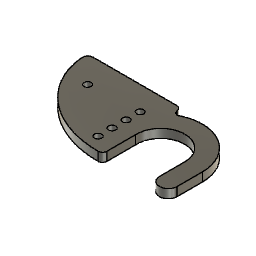
Hook v1 (Autodesk Fusion 360 design; units mm, degrees)
Autodesk Fusion 360 part; units mm, degrees
sketch "Sketch1" plane through (0, 0, 0) normal (0, 0, 1) x (1, 0, 0)
  line L0 (-13.7051, 19.3551) -> (-13.7051, 25.547)
  line L1 (-13.7051, 0.547) -> (-13.7051, -19.453)
  line L2 (-13.7051, -19.453) -> (-105.7051, -19.453)
  line L3 (-13.7051, 25.547) -> (-105.7051, 25.547)
  line L4 (-105.7051, 25.547) -> (-105.7051, -19.453)
  line L5 (13.716, -0.005) -> (13.716, -14.405)
  line L6 (23.716, 0.0066) -> (23.716, -14.3934)
  arc A0 (23.716, 0.0066) -> (-13.7051, 19.3551) centre (0, 0) ccw
  arc A1 (13.716, -0.005) -> (-13.7051, -0.547) centre (0, 0) ccw
  line L7 (13.716, -14.405) -> (23.716, -14.3934)
  circle A2 centre (18.716, -14.3992) radius 5
  dimension "d1" = 27.432
  dimension "d2" = 47.432
  dimension "d4" = 25
  dimension "d5" = 20
  dimension "d6" = 92
  dimension "d7" = 92
  dimension "d8" = 14.4
  dimension "d9" = 14.4
  dimension "d60" = 10
  constraint coincident A0.centre A1.centre
  constraint concentric A0 A1
  constraint coincident L1.start A1
  constraint parallel L0 L1
  constraint perpendicular L1 L2
  constraint perpendicular L0 L3
  constraint vertical L5
  constraint vertical L6
  constraint coincident L1 A1.end
  constraint midpoint L7 A2.centre
  constraint coincident L6.end A2
  measures "d1" diameter of A1
  measures "d2" diameter of A0
  measures "d4" distance of L1.start L0.end
  measures "d5" distance of L1.start L1.end
  measures "d6" distance of L1.end L2.end
  measures "d7" distance of L0.end L3.end
  measures "d8" distance of L5.start L5.end
  measures "d9" distance of L6.start L6.end
  measures "d60" distance of L5 L6
extrude "Extrude1" add sketch "Sketch1" along normal blind 5 contours L7 A2 | L0 L1 L2 L3 L4 L5 L6 A0 A1 A2 picked at (20.2168, -13.6743)
fillet "Fillet1" radius 2 1 edges at (-13.7051, 19.3551, 2.5)
fillet "Fillet2" radius 2.5 1 edges at (-13.7051, 25.547, 2.5)
fillet "Fillet3" radius 2.5 1 edges at (-13.7051, -19.453, 2.5)
fillet "Fillet4" radius 2.5 2 edges at (-105.7051, 25.547, 2.5) (-105.7051, -19.453, 2.5)
sketch "Sketch2" plane through (0, 0, 5) normal (0, 0, 1) x (-1, 0, 0)
  arc A0 (105.7051, 16.953) -> (103.2051, 19.453) centre (103.2051, 16.953) ccw
  line L0 (103.2051, 19.453) -> (16.2051, 19.453)
  arc A1 (16.2051, 19.453) -> (13.7051, 16.953) centre (16.2051, 16.953) ccw
  line L1 (13.7051, 16.953) -> (13.7051, 0.547)
  arc A2 (-13.716, 0.005) -> (13.7051, 0.547) centre (0, 0) ccw
  line L2 (-13.716, 0.005) -> (-13.716, 14.405)
  line L3 (-23.716, 14.3934) -> (-23.716, -0.0066)
  arc A3 (-23.716, -0.0066) -> (10.7948, -21.1169) centre (0, 0) ccw
  arc A4 (13.7051, -22.8977) -> (10.7948, -21.1169) centre (11.7051, -22.8977) ccw
  line L4 (13.7051, -22.8977) -> (13.7051, -23.047)
  arc A5 (13.7051, -23.047) -> (16.2051, -25.547) centre (16.2051, -23.047) ccw
  line L5 (16.2051, -25.547) -> (103.2051, -25.547)
  arc A6 (103.2051, -25.547) -> (105.7051, -23.047) centre (103.2051, -23.047) ccw
  line L6 (105.7051, -23.047) -> (105.7051, 16.953)
  line L7 (0, 0) -> (111.4767, 0) construction
  line L8 (23.7051, -25.547) -> (23.7051, 19.453) construction
  line L9 (59.7051, -25.547) -> (59.7051, 19.453) construction
  line L10 (95.7051, -25.547) -> (95.7051, 19.453) construction
  circle A7 centre (23.7051, 12) radius 2.01
  circle A8 centre (23.7051, 4) radius 2.01
  circle A9 centre (23.7051, -12) radius 2.01
  circle A10 centre (23.7051, -4) radius 2.01
  circle A11 centre (59.7051, 0) radius 2.01
  circle A12 centre (95.7051, 0) radius 2.01
  line L11 (-13.716, 14.405) -> (-23.716, 14.3934)
  dimension "d20" = 10
  dimension "d21" = 36
  dimension "d22" = 36
  dimension "d23" = 4.02
  dimension "d24" = 4.02
  dimension "d26" = 4.02
  dimension "d29" = 4
  dimension "d30" = 8
  dimension "d31" = 4.02
  dimension "d32" = 8
  dimension "d33" = 4
  dimension "d34" = 4.02
  dimension "d35" = 4.02
  constraint coincident A2.centre A3.centre
  constraint perpendicular L6 L7
  constraint coincident L5 L8.start
  constraint coincident L0 L8.end
  constraint perpendicular L0 L8
  constraint coincident L5 L9.start
  constraint coincident L0 L9.end
  constraint perpendicular L0 L9
  constraint coincident L5 L10.start
  constraint coincident L0 L10.end
  constraint perpendicular L0 L10
  constraint coincident L8 A7.centre
  constraint coincident L8 A8.centre
  constraint coincident L8 A9.centre
  constraint coincident L8 A10.centre
  constraint coincident L7 A11.centre
  constraint coincident L9 A11.centre
  constraint coincident L7 A12.centre
  constraint coincident L10 A12.centre
  measures "d20" distance of L1 L8
  measures "d21" distance of L8 L9
  measures "d22" distance of L9 L10
  measures "d23" diameter of A7
  measures "d24" diameter of A8
  measures "d26" diameter of A9
  measures "d29" distance of L7 A8.centre
  measures "d30" distance of A7.centre A8.centre
  measures "d31" diameter of A10
  measures "d32" distance of A9.centre A10.centre
  measures "d33" distance of L7 A10.centre
  measures "d34" diameter of A11
  measures "d35" diameter of A12
extrude "Extrude2" cut sketch "Sketch2" against normal blind 100 contours A7 | A8 | A9 | A10 | A11 | A12
sketch "Sketch3" plane through (0, 0, 5) normal (0, 0, 1) x (-1, 0, 0)
  circle A0 centre (23.7051, -4) radius 2.01
  circle A1 centre (95.7051, 0) radius 2.01
  circle A2 centre (23.7051, 4) radius 2.01
  circle A3 centre (23.7051, -12) radius 2.01
  circle A4 centre (59.7051, 0) radius 2.01
  circle A5 centre (23.7051, 12) radius 2.01
  arc A6 (105.7051, 16.953) -> (103.2051, 19.453) centre (103.2051, 16.953) ccw
  line L0 (103.2051, 19.453) -> (16.2051, 19.453)
  arc A7 (16.2051, 19.453) -> (13.7051, 16.953) centre (16.2051, 16.953) ccw
  line L1 (13.7051, 16.953) -> (13.7051, 0.547)
  arc A8 (-13.716, 0.005) -> (13.7051, 0.547) centre (0, 0) ccw
  line L2 (-13.716, 0.005) -> (-13.716, 14.405)
  line L3 (-23.716, 14.3934) -> (-23.716, -0.0066)
  arc A9 (-23.716, -0.0066) -> (10.7948, -21.1169) centre (0, 0) ccw
  arc A10 (13.7051, -22.8977) -> (10.7948, -21.1169) centre (11.7051, -22.8977) ccw
  line L4 (13.7051, -22.8977) -> (13.7051, -23.047)
  arc A11 (13.7051, -23.047) -> (16.2051, -25.547) centre (16.2051, -23.047) ccw
  line L5 (16.2051, -25.547) -> (103.2051, -25.547)
  arc A12 (103.2051, -25.547) -> (105.7051, -23.047) centre (103.2051, -23.047) ccw
  line L6 (105.7051, -23.047) -> (105.7051, 16.953)
  line L7 (13.7051, -10.547) -> (52.2051, -10.547)
  circle A13 centre (52.2051, -10.547) radius 2.01
  line L8 (52.2051, -10.547) -> (67.2051, -10.547)
  line L9 (67.2051, -10.547) -> (67.2051, -30)
  line L10 (67.2051, -10.547) -> (67.2051, 40.6045)
  ellipse E0 centre (23.7051, 15.4297) end of major axis (68.5434, 15.4297) minor radius 40.9777
  line L11 (-21.1332, 15.4297) -> (68.5434, 15.4297) construction
  line L12 (23.7051, -25.548) -> (23.7051, 56.4074) construction
  line L13 (-13.716, 14.405) -> (-23.716, 14.3934)
  point P0 (67.2051, 0)
  point P1 (25, -25.547)
  dimension "d38" = 38.5
  dimension "d39" = 4.02
  dimension "d55" = 15
  constraint coincident L1 L7.start
  constraint perpendicular L1 L7
  constraint coincident L7.end A13.centre
  constraint parallel L7 L8
  constraint perpendicular L5 L9
  constraint perpendicular L8 L10
  constraint coincident L9 P0
  constraint coincident L5 P1
  constraint coincident E0 L11.start
  constraint coincident E0 L11.end
  constraint coincident E0 L12.start
  constraint coincident E0 L12.end
  constraint perpendicular L10 L11
  measures "d38" distance of L7.start L7.end
  measures "d39" diameter of A13
  measures "d55" distance of L5 L7
extrude "Extrude3" cut sketch "Sketch3" against normal blind 80 contours A6 L0 L5 A12 L6 L9 L10 E0 | L0 L10 E0 picked at (67.4524, 11.238)
sketch "Sketch4" plane through (0, 0, 5) normal (0, 0, 1) x (-1, 0, 0)
  line L0 (50, 5) -> (63.3961, 5)
  line L1 (63.3961, 5) -> (63.3961, -3.8724)
  line L2 (63.3961, -3.8724) -> (50, -3.8724)
  line L3 (50, -3.8724) -> (50, 5)
  constraint horizontal L0
  constraint vertical L1
  constraint horizontal L2
  constraint vertical L3
extrude "Extrude4" add sketch "Sketch3" against normal blind 5 contours A4
extrude "Extrude5" cut sketch "Sketch3" against normal blind 85 contours L7 A13 L8 | L7 A13 L8
sketch "Sketch5" plane through (0, 0, 5) normal (0, 0, 1) x (-1, 0, 0)
  circle A0 centre (52.2051, -10.547) radius 2.01
  line L0 (67.2051, -25.547) -> (67.2051, 19.453)
  line L1 (67.2051, 19.453) -> (16.2051, 19.453)
  arc A1 (16.2051, 19.453) -> (13.7051, 16.953) centre (16.2051, 16.953) ccw
  line L2 (13.7051, 16.953) -> (13.7051, 0.547)
  arc A2 (-13.716, 0.005) -> (13.7051, 0.547) centre (0, 0) ccw
  line L3 (-13.716, 0.005) -> (-13.716, 14.405)
  line L4 (-23.716, 14.3934) -> (-23.716, -0.0066)
  arc A3 (-23.716, -0.0066) -> (10.7948, -21.1169) centre (0, 0) ccw
  arc A4 (13.7051, -22.8977) -> (10.7948, -21.1169) centre (11.7051, -22.8977) ccw
  line L5 (13.7051, -22.8977) -> (13.7051, -23.047)
  arc A5 (13.7051, -23.047) -> (16.2051, -25.547) centre (16.2051, -23.047) ccw
  line L6 (16.2051, -25.547) -> (67.2051, -25.547)
  circle A6 centre (23.7051, 12) radius 2.01
  circle A7 centre (23.7051, -12) radius 2.01
  circle A8 centre (23.7051, 4) radius 2.01
  circle A9 centre (23.7051, -4) radius 2.01
  ellipse E0 centre (16.2051, 19.453) end of major axis (67.2051, 19.453) minor radius 45
  line L7 (-34.7949, 19.453) -> (67.2051, 19.453) construction
  line L8 (16.2051, -25.547) -> (16.2051, 64.453) construction
  line L9 (-13.716, 14.405) -> (-23.716, 14.3934)
  constraint coincident E0 L7.start
  constraint coincident E0 L0.end
  constraint coincident E0 A5.end
  constraint coincident E0 L8.end
  constraint coincident L1.end A1.start
  constraint coincident L0.end L1.start
  constraint coincident A5.end L6.start
sketch "Sketch6" plane through (0, 0, 5) normal (0, 0, 1) x (-1, 0, 0)
  circle A0 centre (52.2051, -10.547) radius 2.01
  line L0 (67.2051, -25.547) -> (67.2051, 19.453)
  line L1 (67.2051, 19.453) -> (16.2051, 19.453)
  arc A1 (16.2051, 19.453) -> (13.7051, 16.953) centre (16.2051, 16.953) ccw
  line L2 (13.7051, 16.953) -> (13.7051, 0.547)
  arc A2 (-13.716, 0.005) -> (13.7051, 0.547) centre (0, 0) ccw
  line L3 (-13.716, 0.005) -> (-13.716, 14.405)
  line L4 (-23.716, 14.3934) -> (-23.716, -0.0066)
  arc A3 (-23.716, -0.0066) -> (10.7948, -21.1169) centre (0, 0) ccw
  arc A4 (13.7051, -22.8977) -> (10.7948, -21.1169) centre (11.7051, -22.8977) ccw
  line L5 (13.7051, -22.8977) -> (13.7051, -23.047)
  arc A5 (13.7051, -23.047) -> (16.2051, -25.547) centre (16.2051, -23.047) ccw
  line L6 (16.2051, -25.547) -> (67.2051, -25.547)
  circle A6 centre (23.7051, 12) radius 2.01
  circle A7 centre (23.7051, -12) radius 2.01
  circle A8 centre (23.7051, 4) radius 2.01
  circle A9 centre (23.7051, -4) radius 2.01
  ellipse E0 centre (16.2051, -25.547) end of major axis (16.2051, 19.453) minor radius 51
  line L7 (16.2051, -70.547) -> (16.2051, 19.453) construction
  line L8 (67.2051, -25.547) -> (-34.7949, -25.547) construction
  line L9 (-13.716, 14.405) -> (-23.716, 14.3934)
  constraint coincident E0 L7.start
  constraint coincident E0 L1.end
  constraint coincident E0 L0.start
  constraint coincident E0 L8.end
  constraint coincident A5.end L6.start
  constraint coincident L1.end A1.start
  constraint coincident L0.start L6.end
extrude "Extrude9" cut sketch "Sketch6" against normal blind 10 contours L0 L1 E0
fillet "Fillet6" radius 3 1 edges at (-67.2051, 25.547, 2.5)
extrude "Extrude10" add sketch "Sketch1" along normal blind 5 contours L7 A2 picked at (20.0461, -16.6414)
